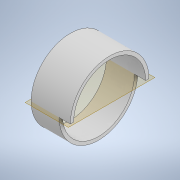
# Autodesk Inventor part: hopper v1
Saved by Autodesk Inventor 2021 (Build 250183000, 183)
## iProperties
Created: 2020-12-01
Part Number: hopper v1
Material: Generic
Document SubType Name: Modeling
Designer: gabe3
Density: 1 g/cm^3
Appearance: Default
Author: gabe3
Autodesk Inventor part; units mm, degrees
ref_plane "YZ Plane" through (0, 0, 0) normal (1, 0, 0) x (0, 1, 0)
ref_plane "XY Plane" through (0, 0, 0) normal (0, 0, 1) x (1, 0, 0)
sketch "Sketch1" plane through (0, 0, 0) normal (1, 0, 0) x (0, 1, 0)
  circle A0 centre (0, 0) radius 69.85
  circle A1 centre (0, 0) radius 76.2
  dimension "d0" = 139.7
  dimension "d1" = 152.4
  constraints: 2 centre point, 2 coincident
  measures "d0" diameter of A0
  measures "d1" diameter of A1
extrude "Extrusion1" add sketch "Sketch1" along normal blind 76.2
sketch "Sketch2" plane through (0, 0, 0) normal (0, 1, 0) x (-1, 0, 0)
  line L0 (-76.2, 76.2) -> (-76.2, -76.2) projected
  line L1 (0, -76.2) -> (-76.2, -76.2) projected
  line L2 (-76.2, 76.2) -> (-54.61, 76.2)
  line L3 (-54.61, 76.2) -> (-54.61, -76.2)
  line L4 (-54.61, -76.2) -> (-76.2, -76.2)
  line L5 (-76.2, -76.2) -> (-76.2, 76.2)
  point P0 (0, 0)
  dimension "d4" = 21.59
  constraints: 8 end point, 2 parallel, 1 horizontal, 1 perpendicular, 1 point on line
  measures "d4" distance of L3.end L4.end
extrude "Extrusion2" cut sketch "Sketch2" against normal blind 76.2
body "Solid1"
